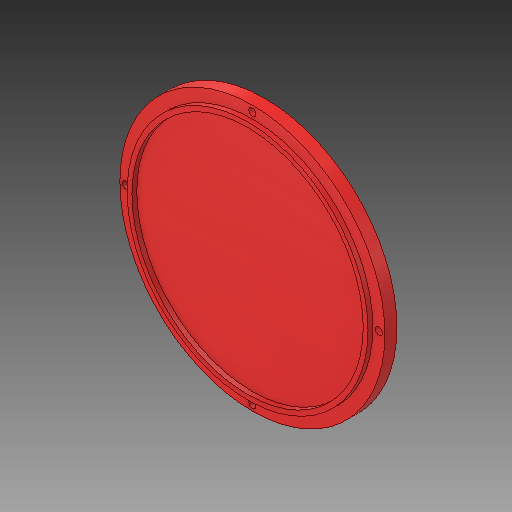
# Autodesk Inventor part: Cover
Saved by Autodesk Inventor 2019 (Build 230136000, 136)
## iProperties
Created: 2022-07-05
Part Number: Cover
Material: Generic
Document SubType Name: Modeling
Designer: zreik
Density: 1 g/cm^3
Appearance: Light Red
Diameter: 110.000 mm
Author: zreik
Autodesk Inventor part; units mm, degrees
ref_plane "YZ Plane" through (0, 0, 0) normal (1, 0, 0) x (0, 1, 0)
ref_plane "XZ Plane" through (0, 0, 0) normal (0, 1, 0) x (-1, 0, 0)
ref_plane "XY Plane" through (0, 0, 0) normal (0, 0, 1) x (1, 0, 0)
sketch "Sketch1" plane through (0, 0, 0) normal (0, 0, 1) x (1, 0, 0)
  circle A0 centre (0, 0) radius 55
  circle A1 centre (0, 0) radius 50
  circle A2 centre (0, 52.5) radius 1.5
  circle A3 centre (-52.5, 0) radius 1.5
  circle A4 centre (0, -52.5) radius 1.5
  circle A5 centre (52.5, 0) radius 1.5
  dimension "d0" = 110
  dimension "d1" = 100
  dimension "d2" = 3
  dimension "d3" = 0
  dimension "d5" = 52.5
  dimension "d8" = 360
  constraints: 6 centre point, 2 coincident, 9 other
  measures "d0" diameter of A0
  measures "d1" diameter of A1
  measures "d2" diameter of A2
  measures "d3" horizontal distance of point (0, 0) A2.centre
  measures "d5" distance of point (0, 0) A2.centre
extrude "Extrusion1" add sketch "Sketch1" along normal blind 5 contours A0 | A1
sketch "Sketch2" plane through (0, 0, 5) normal (0, 0, 1) x (1, 0, 0)
  circle A0 centre (0, 0) radius 50
  circle A1 centre (0, 0) radius 55 projected
  circle A2 centre (0, 0) radius 48
  dimension "d12" = 5
  dimension "d13" = 2
  constraints: 2 centre point, 2 coincident
  measures "d12" radial gap between concentric circles of A1 A0
  measures "d13" radial gap between concentric circles of A0 A2
extrude "Extrusion2" add sketch "Sketch2" along normal blind 2 contours A0
equation "\"d0\" = Diameter"
equation "\"d5\" = 0.25 * d0 + 0.25 * d1"
equation "\"Diameter\" = 110"
body "Solid1"
